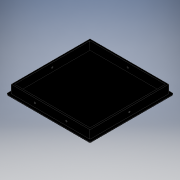
# Autodesk Inventor part: Nanolab CubeDeckel 1
Saved by Autodesk Inventor 2017 (Build 210142000, 142)
## iProperties
Part Number: Nanolab CubeDeckel 1
Material: Generisch
Document SubType Name: Modeling
Designer: David Merges
Density: 1 g/cm^3
Appearance: Eloxiert - schwarz
Author: David Merges
Autodesk Inventor part; units mm, degrees
ref_plane "YZ Plane" through (0, 0, 0) normal (1, 0, 0) x (0, 1, 0)
ref_plane "XZ Plane" through (0, 0, 0) normal (0, 1, 0) x (-1, 0, 0)
ref_plane "XY Plane" through (0, 0, 0) normal (0, 0, 1) x (1, 0, 0)
sketch "Skizze1" plane through (0, 0, 0) normal (0, 0, 1) x (1, 0, 0)
  line L0 (-50.8, 50.8) -> (50.8, 50.8)
  line L1 (50.8, 50.8) -> (50.8, -50.8)
  line L2 (50.8, -50.8) -> (-50.8, -50.8)
  line L3 (-50.8, -50.8) -> (-50.8, 50.8)
  line L4 (50.8, -50.8) -> (-50.8, 50.8) construction
  point P0 (0, 0)
  point P1 (0, 0)
  dimension "d0" = 101.6
  dimension "d1" = 101.6
  constraints: 10 end point, 2 parallel, 1 coincident, 1 horizontal, 1 midpoint, 1 perpendicular
  measures "d0" distance of L1.end L2.end
  measures "d1" distance of L0.end L1.end
extrude "Extrusion1" add sketch "Skizze1" against normal blind 2.0066
fillet "Rundung1" radius 2.0066 4 edges at (50.8, -50.8, -1.0033) (50.8, 50.8, -1.0033) (-50.8, 50.8, -1.0033) (-50.8, -50.8, -1.0033)
fillet "Rundung2" radius 2.0066 8 edges at (-50.2123, -50.2123, -2.0066) (-50.8, 0, -2.0066) (-50.2123, 50.2123, -2.0066) (0, 50.8, -2.0066) (50.2123, 50.2123, -2.0066) (50.8, 0, -2.0066) (50.2123, -50.2123, -2.0066) (0, -50.8, -2.0066)
sketch "Skizze2" plane through (0, 0, 0) normal (0, 0, 1) x (1, 0, 0)
  line L0 (-47.5996, 47.5996) -> (47.5996, 47.5996)
  line L1 (47.5996, 47.5996) -> (47.5996, -47.5996)
  line L2 (47.5996, -47.5996) -> (-47.5996, -47.5996)
  line L3 (-47.5996, -47.5996) -> (-47.5996, 47.5996)
  line L4 (47.5996, -47.5996) -> (-47.5996, 47.5996) construction
  line L5 (-45.593, 45.593) -> (45.593, 45.593)
  line L6 (45.593, 45.593) -> (45.593, -45.593)
  line L7 (45.593, -45.593) -> (-45.593, -45.593)
  line L8 (-45.593, -45.593) -> (-45.593, 45.593)
  line L9 (-45.593, -45.593) -> (45.593, 45.593) construction
  point P0 (0, 0)
  point P1 (0, 0)
  dimension "d6" = 95.1992
  dimension "d7" = 2.0066
  constraints: 20 end point, 4 parallel, 3 perpendicular, 2 horizontal, 2 midpoint, 2 point on line, 1 coincident
  measures "d6" distance of L0.start L0.end
  measures "d7" distance between parallel lines of L1 L6
extrude "Extrusion2" add sketch "Skizze2" along normal blind 9.9822
sketch "Skizze3" plane through (47.5996, -47.5996, 0) normal (1, 0, 0) x (0, 0, -1)
  line L0 (0, 95.1992) -> (0, 0) projected
  line L1 (0, 95.1992) -> (-9.9822, 95.1992) projected
  line L2 (-9.9822, 0) -> (-9.9822, 95.1992) projected
  line L3 (0, 0) -> (-9.9822, 0) projected
  line L4 (0, 47.5996) -> (-4.7752, 47.5996) construction
  line L5 (0, 95.1992) -> (0, 0) construction
  dimension "d10" = 4.7752
  constraints: 2 end point, 1 horizontal, 1 midpoint
  measures "d10" distance of L4.start L4.end
hole "Bohrung1" at (47.5996, 0, 4.7752) direction (-1, 0, 0) diameter 1.941 depth 7.675 tip angle 118 thread size "3-48 UNC" class "2B" standard "ANSI Unified Screw Threads"
pattern_circular "Runde Anordnung1" count 3 over 180 about axis through (0, 0, -10) along (0, 0, 1) of "Bohrung1"
sketch "Skizze4" plane through (-47.5996, -47.5996, 0) normal (0, -1, 0) x (1, 0, 0)
  line L0 (95.1992, 0) -> (0, 0) projected
  line L1 (95.1992, 0) -> (95.1992, 9.9822) projected
  line L2 (0, 9.9822) -> (95.1992, 9.9822) projected
  line L3 (0, 0) -> (0, 9.9822) projected
  line L4 (47.5996, 0) -> (47.5996, 4.7752) construction
  line L5 (28.5496, 4.7752) -> (66.6496, 4.7752) construction
  dimension "d21" = 4.7752
  dimension "d22" = 38.1
  constraints: 4 end point, 1 horizontal, 1 midpoint, 1 vertical
  measures "d21" distance of L4.end L4.start
  measures "d22" distance of L5.start L5.end
hole "Bohrung2" at (-19.05, -47.5996, 4.7752) at (19.05, -47.5996, 4.7752) direction (0, 1, 0) diameter 1.941 depth 7.675 tip angle 118 thread size "3-48 UNC" class "2B" standard "ANSI Unified Screw Threads"
